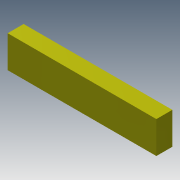
# Autodesk Inventor part: pricna_vystuha1
Saved by Autodesk Inventor 2013 (Build 170138000, 138)
## iProperties
Created: 2013-05-30
Part Number: pricna_vystuha1
Material: Generic
Document SubType Name: Modeling
Designer: idle-rug
Density: 1 g/cm^3
Author: idle-rug
Autodesk Inventor part; units mm, degrees
ref_plane "YZ Plane" through (0, 0, 0) normal (1, 0, 0) x (0, 1, 0)
ref_plane "XZ Plane" through (0, 0, 0) normal (0, 1, 0) x (-1, 0, 0)
ref_plane "XY Plane" through (0, 0, 0) normal (0, 0, 1) x (1, 0, 0)
sketch "Sketch1" plane through (0, 0, 0) normal (0, 1, 0) x (-1, 0, 0)
  line L0 (46.5, 10) -> (-46.5, 10)
  line L1 (-46.5, 10) -> (-46.5, -10)
  line L2 (-46.5, -10) -> (46.5, -10)
  line L3 (46.5, -10) -> (46.5, 10)
  line L4 (46.5, 10) -> (-46.5, -10) construction
  line L5 (-46.5, 10) -> (46.5, -10) construction
  point P0 (0, 0)
  dimension "d0" = 93
  dimension "d1" = 20
  constraints: 12 end point, 2 midpoint, 2 parallel, 1 horizontal, 1 perpendicular
  measures "d0" distance of L2.end L1.end
  measures "d1" distance of L1.end L0.end
extrude "Extrusion1" add sketch "Sketch1" along normal blind 10
body "Solid1"
